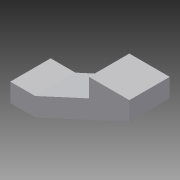
# Autodesk Inventor part: hph_B_001
Saved by Autodesk Inventor 2014 (Build 180170000, 170)
## iProperties
Created: 2014-03-22
Part Number: hph_B_001
Material: Generic
Document SubType Name: Modeling
Designer: stephenholtz
Density: 1 g/cm^3
Appearance: Default
Mass: 4.83942 g
Surface Area: 26.7447 cm^2
Volume: 4.83942 cm^3
Description: CNC 302 Stainless Steel
Author: stephenholtz
Revision Number: 1
Autodesk Inventor part; units mm, degrees
ref_plane "YZ Plane" through (0, 0, 0) normal (1, 0, 0) x (0, 1, 0)
ref_plane "XZ Plane" through (0, 0, 0) normal (0, 1, 0) x (-1, 0, 0)
ref_plane "XY Plane" through (0, 0, 0) normal (0, 0, 1) x (1, 0, 0)
sketch "Sketch1" plane through (0, 0, 0) normal (0, 0, 1) x (1, 0, 0)
  line L0 (3.81, -5.08) -> (-3.81, -5.08)
  line L1 (-3.81, -5.08) -> (-3.81, 5.08)
  line L2 (-3.81, 5.08) -> (3.81, 5.08)
  line L3 (3.81, 5.08) -> (3.81, -5.08)
  line L4 (3.81, -5.08) -> (-3.81, 5.08) construction
  line L5 (-3.81, -5.08) -> (3.81, 5.08) construction
  line L6 (-13.97, -27.0933) -> (-21.59, -27.0933)
  line L7 (-21.59, -27.0933) -> (-21.59, -43.6033)
  line L8 (-21.59, -43.6033) -> (-13.97, -43.6033)
  line L9 (-13.97, -43.6033) -> (-13.97, -27.0933)
  line L10 (-13.97, -27.0933) -> (-3.81, -5.08)
  line L11 (-13.97, -43.6033) -> (3.81, -5.08)
  point P0 (0, 0)
  dimension "contact_rec_len" = 10.16
  dimension "contact_rec_offset" = 7.62
  dimension "d3" = 7.62
  dimension "d4" = 16.51
  dimension "d39" = 25.4
  constraints: 24 end point, 6 parallel, 2 midpoint, 2 perpendicular, 1 horizontal
  measures "contact_rec_len" distance of L2.end L0.start
  measures "contact_rec_offset" distance of L1.end L2.end
  measures "d3" distance of L7.end L8.end
  measures "d4" distance of L6.end L7.end
  measures "d39" distance between parallel lines of L3 L7
extrude "Extrusion2" add sketch "Sketch1" along normal blind 16.51
sketch "Sketch3" plane through (-21.59, -43.2093, 0) normal (-1, 0, 0) x (0, 0, 1)
  line L0 (0, 12.7) -> (0, 0) construction
  line L1 (0, 0) -> (12.7, 0) construction
  line L2 (12.7, 12.7) -> (12.7, 0) construction
  line L3 (0, 12.7) -> (12.7, 12.7) construction
  line L4 (6.35, 0) -> (6.35, 12.7) construction
  line L5 (9.525, 0) -> (9.525, 12.7) construction
  line L6 (3.175, 0) -> (3.175, 12.7) construction
  line L7 (6.35, 0) -> (6.35, 12.7) construction
  line L8 (12.7, 6.35) -> (0, 6.35) construction
  point P0 (0, 43.2093)
  point P1 (9.525, 6.35)
  point P2 (3.175, 6.35)
  dimension "d10" = 4.1275
  dimension "d13" = 4.1275
  dimension "d66" = 6.35
  constraints: 10 end point, 6 midpoint, 2 horizontal, 2 point on line, 1 perpendicular, 9 other
  measures "d66" distance between parallel lines of L1 L8
sketch "Sketch6" plane through (-3.81, -5.08, 0) normal (-1, 0, 0) x (0, 0, 1)
  line L0 (0, 10.16) -> (0, 0) construction
  line L1 (0, 0) -> (12.7, 0) construction
  line L2 (12.7, 10.16) -> (12.7, 0) construction
  line L3 (0, 10.16) -> (12.7, 10.16) construction
  line L4 (6.35, 10.16) -> (6.35, 0) construction
  line L5 (9.525, 10.16) -> (9.525, 0) construction
  line L6 (3.175, 10.16) -> (3.175, 0) construction
  line L7 (6.35, 10.16) -> (6.35, 0) construction
  point P0 (0, 5.08)
  point P1 (9.525, 5.08)
  point P2 (3.175, 5.08)
  dimension "d49" = 4.1275
  dimension "d52" = 4.1275
  constraints: 8 end point, 4 midpoint, 2 horizontal, 9 other
equation "\"d3\" = contact_rec_offset"
equation "\"d74\" = 2 * hole_spacing"
equation "\"d10\" = 0.5 * hole_spacing"
equation "\"d13\" = 0.5 * hole_spacing"
equation "\"d49\" = 0.5 * hole_spacing"
equation "\"d52\" = 0.5 * hole_spacing"
equation "\"hole_spacing\" = 8.255"
equation "\"d46\" = 6.35"
body "Solid1"
body "Solid2"
